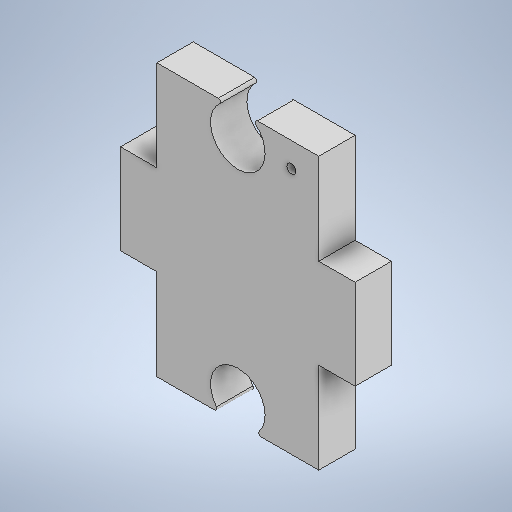
# Autodesk Inventor part: Spacer
Saved by Autodesk Inventor 2025.1 (Build 291241000, 241)
## iProperties
Created: 2025-03-30
Part Number: Spacer
Material: Všeobecné
Document SubType Name: Modeling
Designer: 42060
Density: 1 g/cm^3
Appearance: Výchozí
Author: 42060
Autodesk Inventor part; units mm, degrees
ref_plane "YZ Plane" through (0, 0, 0) normal (1, 0, 0) x (0, 1, 0)
ref_plane "XZ Plane" through (0, 0, 0) normal (0, 1, 0) x (-1, 0, 0)
ref_plane "XY Plane" through (0, 0, 0) normal (0, 0, 1) x (1, 0, 0)
sketch "Náčrt1" plane through (0, 0, 0) normal (0, 0, 1) x (1, 0, 0)
  line L0 (-8.9, 4.95) -> (-8.9, 14.95)
  line L1 (-8.9, 14.95) -> (-2.15, 14.95)
  line L2 (2.15, 14.95) -> (8.9, 14.95)
  line L3 (8.9, 14.95) -> (8.9, 4.95)
  line L4 (8.9, 4.95) -> (12.9, 4.95)
  line L5 (12.9, 4.95) -> (12.9, -4.95)
  line L6 (12.9, -4.95) -> (8.9, -4.95)
  line L7 (8.9, -4.95) -> (8.9, -14.95)
  line L8 (-8.9, -14.95) -> (-8.9, -4.95)
  line L9 (-12.9, -4.95) -> (-12.9, 4.95)
  line L10 (-12.9, 4.95) -> (-8.9, 4.95)
  line L11 (-8.9, -4.95) -> (-12.9, -4.95)
  arc A0 (-1.9846, 14.5125) -> (1.9846, 14.5125) centre (0, 12.2628) ccw
  arc A1 (-1.9846, 14.5125) -> (-2.15, 14.95) centre (-2.15, 14.7) ccw
  arc A2 (2.15, 14.95) -> (1.9846, 14.5125) centre (2.15, 14.7) ccw
  line L12 (-8.9, -14.95) -> (-2.5458, -14.95)
  arc A3 (2.35, -14.5446) -> (-2.35, -14.5446) centre (0, -12.6798) ccw
  line L13 (2.5458, -14.95) -> (8.9, -14.95)
  arc A4 (-2.5458, -14.95) -> (-2.35, -14.5446) centre (-2.5458, -14.7) ccw
  arc A5 (2.35, -14.5446) -> (2.5458, -14.95) centre (2.5458, -14.7) ccw
  circle A6 centre (5.9, 12.2628) radius 0.5
  point P0 (0, 0)
  point P1 (-1.3338, 14.95)
  point P2 (1.3338, 14.95)
  point P3 (12.9, 0)
  point P4 (-1.9612, -14.95)
  point P5 (1.9612, -14.95)
  dimension "d0" = 9.9
  dimension "d1" = 17.8
  dimension "d2" = 4
  dimension "d4" = 3
  dimension "d5" = 0.25
  dimension "d6" = 3.8
  dimension "d7" = 0.25
  dimension "d8" = 4.7
  dimension "d18" = 1
  dimension "d19" = 3
  dimension "d20" = 10
  constraints: 28 end point, 16 point on circle, 12 point on line, 8 tangent, 7 centre point, 6 perpendicular, 4 equal length, 3 equal radius, 3 horizontal, 3 horizontal alignment, 2 vertical, 2 vertical alignment, 1 midpoint
  measures "d0" distance of L4.end L5.end
  measures "d1" distance of L7.end L8.start
  measures "d2" distance of L5.end L6.end
  measures "d4" radius of A0
  measures "d5" radius of A1
  measures "d7" radius of A4
  measures "d8" distance of A3.start A3.end
  measures "d18" diameter of A6
  measures "d19" distance from line of L3 A6.centre
  measures "d20" distance of L2.end L3.end
extrude "Vysunutí1" add sketch "Náčrt1" along normal mid plane 4
